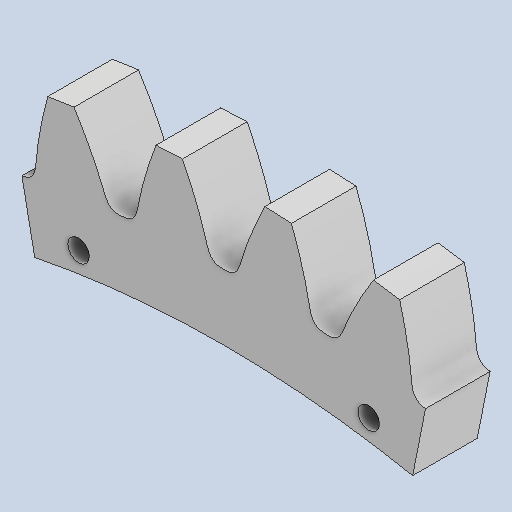
# Autodesk Inventor part: sector big gear
Saved by Autodesk Inventor 2025 (Build 290162010, 162A)
## iProperties
Created: 2025-08-27
Part Number: sector big gear
Material: Generic
Document SubType Name: Modeling
Designer: pokla
Density: 1 g/cm^3
Appearance: Default
Author: pokla
Autodesk Inventor part; units mm, degrees
(part 1 of 2)
ref_plane "YZ Plane" through (0, 0, 0) normal (1, 0, 0) x (0, 1, 0)
ref_plane "XZ Plane" through (0, 0, 0) normal (0, 1, 0) x (-1, 0, 0)
ref_plane "XY Plane" through (0, 0, 0) normal (0, 0, 1) x (1, 0, 0)
sketch "Sketch1" plane through (0, 0, 0) normal (0, 0, 1) x (1, 0, 0)
  spline S0 degree 3 poles (-15.3136, 412.2157) (-14.7005, 410.9627) (-13.4744, 408.4567) (-11.7613, 404.6382) (-10.1461, 400.7772) (-8.6557, 396.867) (-7.2691, 392.9165) (-6.406, 389.9001) (-5.7884, 387.899) (-5.3377, 386.951) (-4.8395, 386.2299) (-4.359, 385.7235) (-3.8332, 385.2647) (-3.236, 384.8928) (-2.5894, 384.6288) (-2.0848, 384.4891) (-1.5698, 384.3899) (-0.8714, 384.3654) (0, 384.3814) (0.8714, 384.3654) (1.5698, 384.3899) (2.0848, 384.4891) (2.5894, 384.6288) (3.236, 384.8928) (3.8332, 385.2647) (4.359, 385.7235) (4.8395, 386.2299) (5.3377, 386.951) (5.7884, 387.899) (6.406, 389.9001) (7.2691, 392.9165) (8.6557, 396.867) (10.1461, 400.7772) (11.7613, 404.6382) (13.4744, 408.4567) (14.7005, 410.9627) (15.3136, 412.2157) knots 0 0 0 0 0.418453 0.836906 1.255357 1.673806 2.09225 2.510695 2.615288 2.719831 2.824322 2.876636 2.92893 3.033403 3.085707 3.138007 3.190298 3.242598 3.347213 3.451829 3.504129 3.55642 3.60872 3.661023 3.765497 3.817791 3.870105 3.974596 4.079139 4.183732 4.602176 5.020621 5.43907 5.857521 6.275974 6.694427 6.694427 6.694427 6.694427
  circle A0 centre (0, 0) radius 384.375 construction
  circle A1 centre (0, 0) radius 375.877 construction
  circle A2 centre (0, 0) radius 400 construction
  circle A3 centre (0, 0) radius 412.5
  point P0 (-13.4954, 408.4468)
  point P1 (-11.7776, 404.6311)
  point P2 (-10.1669, 400.769)
  point P3 (-8.673, 396.8603)
  point P4 (-7.3084, 392.9046)
  point P5 (-6.0957, 388.8997)
  point P6 (-5.7647, 387.9075)
  point P7 (-5.3131, 386.9647)
  point P8 (-4.7127, 386.1094)
  point P9 (-4.3533, 385.7294)
  point P10 (-3.9585, 385.3864)
  point P11 (-3.0706, 384.8359)
  point P12 (-2.5862, 384.6385)
  point P13 (-2.083, 384.4958)
  point P14 (-1.5684, 384.4034)
  point P15 (-1.0462, 384.3746)
  point P16 (0, 384.375)
  point P17 (1.0462, 384.3746)
  point P18 (1.5684, 384.4034)
  point P19 (2.083, 384.4958)
  point P20 (2.5862, 384.6385)
  point P21 (3.0706, 384.8359)
  point P22 (3.9585, 385.3864)
  point P23 (4.3533, 385.7294)
  point P24 (4.7127, 386.1094)
  point P25 (5.3131, 386.9647)
  point P26 (5.7647, 387.9075)
  point P27 (6.0957, 388.8997)
  point P28 (7.3084, 392.9046)
  point P29 (8.673, 396.8603)
  point P30 (10.1669, 400.769)
  point P31 (11.7776, 404.6311)
  point P32 (13.4954, 408.4468)
  constraints: 4 centre point, 2 point on circle, 75 other
extrude "Extrusion1" add sketch "Sketch1" against normal blind 24
extrude "Extrusion2" cut sketch "Sketch1" against normal through all contours A3 S0 picked at (-1.5801, 403.5429)
pattern_circular "Circular Pattern1" count 64 over 360 about axis through (0, 0, -10) along (0, 0, 1) of "Extrusion2"
sketch "Sketch2" plane through (0, 0, 0) normal (0, 0, 1) x (1, 0, 0)
  arc A0 (25.1644, 411.7317) -> (15.3136, 412.2157) centre (0, 0) ccw projected
  arc A1 (-15.3136, 412.2157) -> (-25.1644, 411.7317) centre (0, 0) ccw projected
  arc A2 (-55.644, 408.7297) -> (-65.4, 407.2826) centre (0, 0) ccw projected
  spline S0 degree 3 poles (-65.4, 407.2826) (-65.7568, 405.9341) (-66.4705, 403.237) (-67.4057, 399.1577) (-68.2366, 395.0558) (-68.9355, 390.9299) (-69.5247, 386.7848) (-69.7828, 383.658) (-69.9982, 381.5749) (-70.2552, 380.5572) (-70.6032, 379.7528) (-70.9757, 379.1623) (-71.4018, 378.6098) (-71.915, 378.1285) (-72.4977, 377.7435) (-72.9654, 377.508) (-73.4511, 377.3102) (-74.1313, 377.1499) (-74.9891, 376.9957) (-75.8406, 376.8099) (-76.5304, 376.6977) (-77.0548, 376.6945) (-77.5771, 376.7331) (-78.2627, 376.8658) (-78.921, 377.1141) (-79.5261, 377.4615) (-80.0962, 377.8645) (-80.7256, 378.4745) (-81.3525, 379.3164) (-82.3487, 381.1585) (-83.7837, 383.9485) (-85.9143, 387.5526) (-88.1389, 391.097) (-90.4763, 394.5686) (-92.9014, 397.9796) (-94.5929, 400.1982) (-95.4386, 401.3075) knots 0 0 0 0 0.062508 0.125015 0.187523 0.25003 0.312536 0.375043 0.390666 0.406283 0.421892 0.429706 0.437518 0.453124 0.460937 0.468749 0.47656 0.484373 0.5 0.515627 0.52344 0.531251 0.539063 0.546876 0.562482 0.570294 0.578108 0.593717 0.609334 0.624957 0.687464 0.74997 0.812477 0.874985 0.937492 1 1 1 1 projected
  arc A3 (-95.4386, 401.3075) -> (-105.0057, 398.9111) centre (0, 0) ccw projected
  spline S1 degree 3 poles (-105.0057, 398.9111) (-105.2286, 397.5341) (-105.6745, 394.7801) (-106.2054, 390.6287) (-106.6303, 386.4651) (-106.9214, 382.2906) (-107.1015, 378.1077) (-107.0519, 374.9707) (-107.062, 372.8765) (-107.2181, 371.8385) (-107.4855, 371.0038) (-107.7983, 370.3797) (-108.1683, 369.7881) (-108.6318, 369.2588) (-109.1739, 368.8185) (-109.6163, 368.5383) (-110.0803, 368.2939) (-110.7415, 368.0677) (-111.58, 367.8301) (-112.4092, 367.5618) (-113.0847, 367.3825) (-113.6063, 367.3279) (-114.1298, 367.3152) (-114.8251, 367.38) (-115.5046, 367.5626) (-116.1409, 367.849) (-116.7477, 368.1942) (-117.4338, 368.7396) (-118.1403, 369.5159) (-119.3122, 371.2516) (-121.0137, 373.8875) (-123.4874, 377.2654) (-126.0487, 380.5746) (-128.7151, 383.8005) (-131.4629, 386.9573) (-133.3637, 388.9994) (-134.3141, 390.0205) knots 0 0 0 0 0.062508 0.125015 0.187523 0.25003 0.312536 0.375043 0.390666 0.406283 0.421892 0.429706 0.437518 0.453124 0.460937 0.468749 0.47656 0.484373 0.5 0.515627 0.52344 0.531251 0.539063 0.546876 0.562482 0.570294 0.578108 0.593717 0.609334 0.624957 0.687464 0.74997 0.812477 0.874985 0.937492 1 1 1 1 projected
  arc A4 (-134.3141, 390.0205) -> (-143.6002, 386.6979) centre (0, 0) ccw projected
  spline S2 degree 3 poles (-143.6002, 386.6979) (-143.6871, 385.3056) (-143.8609, 382.5212) (-143.9823, 378.3378) (-143.9971, 374.1526) (-143.8776, 369.9697) (-143.6468, 365.7892) (-143.2899, 362.6722) (-143.0948, 360.5871) (-143.1483, 359.5388) (-143.3327, 358.6819) (-143.5828, 358.0301) (-143.893, 357.4051) (-144.3024, 356.8329) (-144.7987, 356.3416) (-145.2115, 356.0194) (-145.6494, 355.7307) (-146.2852, 355.4408) (-147.0964, 355.1221) (-147.8953, 354.7738) (-148.55, 354.5292) (-149.0637, 354.4238) (-149.5834, 354.3598) (-150.2818, 354.3562) (-150.9759, 354.4713) (-151.6371, 354.6939) (-152.2749, 354.9779) (-153.0112, 355.4535) (-153.7903, 356.1568) (-155.1267, 357.7693) (-157.0784, 360.2257) (-159.8713, 363.3449) (-162.7446, 366.3871) (-165.7143, 369.3361) (-168.7583, 372.2083) (-170.8501, 374.0544) (-171.896, 374.9774) knots 0 0 0 0 0.062508 0.125015 0.187523 0.25003 0.312536 0.375043 0.390666 0.406283 0.421892 0.429706 0.437518 0.453124 0.460937 0.468749 0.47656 0.484373 0.5 0.515627 0.52344 0.531251 0.539063 0.546876 0.562482 0.570294 0.578108 0.593717 0.609334 0.624957 0.687464 0.74997 0.812477 0.874985 0.937492 1 1 1 1 projected
  arc A5 (-171.896, 374.9774) -> (-180.8117, 370.7605) centre (0, 0) ccw projected
  spline S3 degree 3 poles (-180.8117, 370.7605) (-180.7618, 369.3665) (-180.6618, 366.5784) (-180.3726, 362.4032) (-179.977, 358.2368) (-179.4481, 354.0857) (-178.8087, 349.948) (-178.1481, 346.881) (-177.7494, 344.825) (-177.7, 343.7765) (-177.7995, 342.9057) (-177.9845, 342.2325) (-178.2319, 341.5801) (-178.5833, 340.9705) (-179.0291, 340.433) (-179.4083, 340.0719) (-179.8157, 339.7416) (-180.4201, 339.3908) (-181.1962, 338.9942) (-181.9571, 338.5692) (-182.5846, 338.2616) (-183.0855, 338.1063) (-183.5965, 337.9917) (-184.2911, 337.9197) (-184.9931, 337.9662) (-185.673, 338.1229) (-186.3356, 338.3431) (-187.1149, 338.7442) (-187.9592, 339.3678) (-189.4472, 340.8414) (-191.6303, 343.0947) (-194.7155, 345.9252) (-197.8731, 348.6711) (-201.1176, 351.3148) (-204.4285, 353.8749) (-206.6912, 355.5069) (-207.8225, 356.323) knots 0 0 0 0 0.062508 0.125015 0.187523 0.25003 0.312536 0.375043 0.390666 0.406283 0.421892 0.429706 0.437518 0.453124 0.460937 0.468749 0.47656 0.484373 0.5 0.515627 0.52344 0.531251 0.539063 0.546876 0.562482 0.570294 0.578108 0.593717 0.609334 0.624957 0.687464 0.74997 0.812477 0.874985 0.937492 1 1 1 1 projected
  arc A6 (-207.8225, 356.323) -> (-216.282, 351.2526) centre (0, 0) ccw projected
  spline S4 degree 3 poles (-216.282, 351.2526) (-216.0956, 349.8701) (-215.7228, 347.1053) (-215.0258, 342.9785) (-214.2237, 338.8709) (-213.2905, 334.7917) (-212.2486, 330.7366) (-211.2905, 327.7491) (-210.6923, 325.7421) (-210.5403, 324.7035) (-210.554, 323.8271) (-210.6721, 323.139) (-210.8544, 322.4655) (-211.1443, 321.8245) (-211.5353, 321.2458) (-211.8773, 320.8492) (-212.2504, 320.4807) (-212.8174, 320.0722) (-213.5509, 319.6015) (-214.2665, 319.104) (-214.8608, 318.7364) (-215.3441, 318.5327) (-215.8414, 318.3686) (-216.5256, 318.2288) (-217.2288, 318.2063) (-217.9208, 318.2956) (-218.6017, 318.4498) (-219.4166, 318.7725) (-220.318, 319.3104) (-221.9433, 320.6311) (-224.3367, 322.6596) (-227.6844, 325.174) (-231.096, 327.5972) (-234.5841, 329.9101) (-238.1299, 332.1334) (-240.5417, 333.5358) (-241.7475, 334.237) knots 0 0 0 0 0.062508 0.125015 0.187523 0.25003 0.312536 0.375043 0.390666 0.406283 0.421892 0.429706 0.437518 0.453124 0.460937 0.468749 0.47656 0.484373 0.5 0.515627 0.52344 0.531251 0.539063 0.546876 0.562482 0.570294 0.578108 0.593717 0.609334 0.624957 0.687464 0.74997 0.812477 0.874985 0.937492 1 1 1 1 projected
  arc A7 (-241.7475, 334.237) -> (-249.6693, 328.3618) centre (0, 0) ccw projected
  spline S5 degree 3 poles (-249.6693, 328.3618) (-249.3483, 327.0043) (-248.7063, 324.2894) (-247.6081, 320.2508) (-246.4074, 316.2416) (-245.0788, 312.2735) (-243.6444, 308.34) (-242.3981, 305.4608) (-241.6061, 303.5221) (-241.353, 302.5034) (-241.2807, 301.6299) (-241.3308, 300.9336) (-241.4462, 300.2454) (-241.6719, 299.579) (-242.0043, 298.9648) (-242.3057, 298.5367) (-242.6409, 298.1333) (-243.1652, 297.6712) (-243.849, 297.1309) (-244.5124, 296.5656) (-245.0678, 296.1416) (-245.5289, 295.8915) (-246.0076, 295.6794) (-246.6748, 295.4732) (-247.3725, 295.3819) (-248.0699, 295.403) (-248.7627, 295.4896) (-249.6053, 295.731) (-250.555, 296.1779) (-252.3019, 297.3329) (-254.8827, 299.117) (-258.4607, 301.2912) (-262.0934, 303.3684) (-265.7913, 305.3283) (-269.538, 307.1932) (-272.0756, 308.3525) (-273.3444, 308.9322) knots 0 0 0 0 0.062508 0.125015 0.187523 0.25003 0.312536 0.375043 0.390666 0.406283 0.421892 0.429706 0.437518 0.453124 0.460937 0.468749 0.47656 0.484373 0.5 0.515627 0.52344 0.531251 0.539063 0.546876 0.562482 0.570294 0.578108 0.593717 0.609334 0.624957 0.687464 0.74997 0.812477 0.874985 0.937492 1 1 1 1 projected
  arc A8 (-273.3444, 308.9322) -> (-280.6521, 302.3088) centre (0, 0) ccw projected
  spline S6 degree 3 poles (-280.6521, 302.3088) (-280.1997, 300.9893) (-279.2947, 298.3503) (-277.8059, 294.4389) (-276.2179, 290.5667) (-274.5068, 286.7478) (-272.6938, 282.9739) (-271.1713, 280.2307) (-270.193, 278.379) (-269.8414, 277.39) (-269.6838, 276.5278) (-269.6654, 275.8299) (-269.7128, 275.1338) (-269.8721, 274.4485) (-270.1426, 273.8047) (-270.4007, 273.349) (-270.6947, 272.9147) (-271.1712, 272.4035) (-271.7987, 271.7987) (-272.4035, 271.1712) (-272.9147, 270.6947) (-273.349, 270.4007) (-273.8047, 270.1426) (-274.4485, 269.8721) (-275.1338, 269.7128) (-275.8299, 269.6654) (-276.5278, 269.6838) (-277.39, 269.8414) (-278.379, 270.193) (-280.2307, 271.1713) (-282.9739, 272.6938) (-286.7478, 274.5068) (-290.5667, 276.2179) (-294.4389, 277.8059) (-298.3503, 279.2947) (-300.9893, 280.1997) (-302.3088, 280.6521) knots 0 0 0 0 0.062508 0.125015 0.187523 0.25003 0.312536 0.375043 0.390666 0.406283 0.421892 0.429706 0.437518 0.453124 0.460937 0.468749 0.47656 0.484373 0.5 0.515627 0.52344 0.531251 0.539063 0.546876 0.562482 0.570294 0.578108 0.593717 0.609334 0.624957 0.687464 0.74997 0.812477 0.874985 0.937492 1 1 1 1 projected
  arc A9 (-302.3088, 280.6521) -> (-308.9322, 273.3444) centre (0, 0) ccw projected
  spline S7 degree 3 poles (-308.9322, 273.3444) (-308.3525, 272.0756) (-307.1932, 269.538) (-305.3283, 265.7913) (-303.3684, 262.0934) (-301.2912, 258.4607) (-299.117, 254.8827) (-297.3329, 252.3019) (-296.1779, 250.555) (-295.731, 249.6053) (-295.4896, 248.7627) (-295.403, 248.0699) (-295.3819, 247.3725) (-295.4732, 246.6748) (-295.6794, 246.0076) (-295.8915, 245.5289) (-296.1416, 245.0678) (-296.5656, 244.5124) (-297.1309, 243.849) (-297.6712, 243.1652) (-298.1333, 242.6409) (-298.5367, 242.3057) (-298.9648, 242.0043) (-299.579, 241.6719) (-300.2454, 241.4462) (-300.9336, 241.3308) (-301.6299, 241.2807) (-302.5034, 241.353) (-303.5221, 241.6061) (-305.4608, 242.3981) (-308.34, 243.6444) (-312.2735, 245.0788) (-316.2416, 246.4074) (-320.2508, 247.6081) (-324.2894, 248.7063) (-327.0043, 249.3483) (-328.3618, 249.6693) knots 0 0 0 0 0.062508 0.125015 0.187523 0.25003 0.312536 0.375043 0.390666 0.406283 0.421892 0.429706 0.437518 0.453124 0.460937 0.468749 0.47656 0.484373 0.5 0.515627 0.52344 0.531251 0.539063 0.546876 0.562482 0.570294 0.578108 0.593717 0.609334 0.624957 0.687464 0.74997 0.812477 0.874985 0.937492 1 1 1 1 projected
  arc A10 (-328.3618, 249.6693) -> (-334.237, 241.7475) centre (0, 0) ccw projected
  spline S8 degree 3 poles (-334.237, 241.7475) (-333.5358, 240.5417) (-332.1334, 238.1299) (-329.9101, 234.5841) (-327.5972, 231.096) (-325.174, 227.6844) (-322.6596, 224.3367) (-320.6311, 221.9433) (-319.3104, 220.318) (-318.7725, 219.4166) (-318.4498, 218.6017) (-318.2956, 217.9208) (-318.2063, 217.2288) (-318.2288, 216.5256) (-318.3686, 215.8414) (-318.5327, 215.3441) (-318.7364, 214.8608) (-319.104, 214.2665) (-319.6015, 213.5509) (-320.0722, 212.8174) (-320.4807, 212.2504) (-320.8492, 211.8773) (-321.2458, 211.5353) (-321.8245, 211.1443) (-322.4655, 210.8544) (-323.139, 210.6721) (-323.8271, 210.554) (-324.7035, 210.5403) (-325.7421, 210.6923) (-327.7491, 211.2905) (-330.7366, 212.2486) (-334.7917, 213.2905) (-338.8709, 214.2237) (-342.9785, 215.0258) (-347.1053, 215.7228) (-349.8701, 216.0956) (-351.2526, 216.282) knots 0 0 0 0 0.062508 0.125015 0.187523 0.25003 0.312536 0.375043 0.390666 0.406283 0.421892 0.429706 0.437518 0.453124 0.460937 0.468749 0.47656 0.484373 0.5 0.515627 0.52344 0.531251 0.539063 0.546876 0.562482 0.570294 0.578108 0.593717 0.609334 0.624957 0.687464 0.74997 0.812477 0.874985 0.937492 1 1 1 1 projected
  arc A11 (-351.2526, 216.282) -> (-356.323, 207.8225) centre (0, 0) ccw projected
  spline S9 degree 3 poles (-356.323, 207.8225) (-355.5069, 206.6912) (-353.8749, 204.4285) (-351.3148, 201.1176) (-348.6711, 197.8731) (-345.9252, 194.7155) (-343.0947, 191.6303) (-340.8414, 189.4472) (-339.3678, 187.9592) (-338.7442, 187.1149) (-338.3431, 186.3356) (-338.1229, 185.673) (-337.9662, 184.9931) (-337.9197, 184.2911) (-337.9917, 183.5965) (-338.1063, 183.0855) (-338.2616, 182.5846) (-338.5692, 181.9571) (-338.9942, 181.1962) (-339.3908, 180.4201) (-339.7416, 179.8157) (-340.0719, 179.4083) (-340.433, 179.0291) (-340.9705, 178.5833) (-341.5801, 178.2319) (-342.2325, 177.9845) (-342.9057, 177.7995) (-343.7765, 177.7) (-344.825, 177.7494) (-346.881, 178.1481) (-349.948, 178.8087) (-354.0857, 179.4481) (-358.2368, 179.977) (-362.4032, 180.3726) (-366.5784, 180.6618) (-369.3665, 180.7618) (-370.7605, 180.8117) knots 0 0 0 0 0.062508 0.125015 0.187523 0.25003 0.312536 0.375043 0.390666 0.406283 0.421892 0.429706 0.437518 0.453124 0.460937 0.468749 0.47656 0.484373 0.5 0.515627 0.52344 0.531251 0.539063 0.546876 0.562482 0.570294 0.578108 0.593717 0.609334 0.624957 0.687464 0.74997 0.812477 0.874985 0.937492 1 1 1 1 projected
  arc A12 (-370.7605, 180.8117) -> (-374.9774, 171.896) centre (0, 0) ccw projected
  spline S10 degree 3 poles (-374.9774, 171.896) (-374.0544, 170.8501) (-372.2083, 168.7583) (-369.3361, 165.7143) (-366.3871, 162.7446) (-363.3449, 159.8713) (-360.2257, 157.0784) (-357.7693, 155.1267) (-356.1568, 153.7903) (-355.4535, 153.0112) (-354.9779, 152.2749) (-354.6939, 151.6371) (-354.4713, 150.9759) (-354.3562, 150.2818) (-354.3598, 149.5834) (-354.4238, 149.0637) (-354.5292, 148.55) (-354.7738, 147.8953) (-355.1221, 147.0964) (-355.4408, 146.2852) (-355.7307, 145.6494) (-356.0194, 145.2115) (-356.3416, 144.7987) (-356.8329, 144.3024) (-357.4051, 143.893) (-358.0301, 143.5828) (-358.6819, 143.3327) (-359.5388, 143.1483) (-360.5871, 143.0948) (-362.6722, 143.2899) (-365.7892, 143.6468) (-369.9697, 143.8776) (-374.1526, 143.9971) (-378.3378, 143.9823) (-382.5212, 143.8609) (-385.3056, 143.6871) (-386.6979, 143.6002) knots 0 0 0 0 0.062508 0.125015 0.187523 0.25003 0.312536 0.375043 0.390666 0.406283 0.421892 0.429706 0.437518 0.453124 0.460937 0.468749 0.47656 0.484373 0.5 0.515627 0.52344 0.531251 0.539063 0.546876 0.562482 0.570294 0.578108 0.593717 0.609334 0.624957 0.687464 0.74997 0.812477 0.874985 0.937492 1 1 1 1 projected
  arc A13 (-386.6979, 143.6002) -> (-390.0205, 134.3141) centre (0, 0) ccw projected
  spline S11 degree 3 poles (-390.0205, 134.3141) (-388.9994, 133.3637) (-386.9573, 131.4629) (-383.8005, 128.7151) (-380.5746, 126.0487) (-377.2654, 123.4874) (-373.8875, 121.0137) (-371.2516, 119.3122) (-369.5159, 118.1403) (-368.7396, 117.4338) (-368.1942, 116.7477) (-367.849, 116.1409) (-367.5626, 115.5046) (-367.38, 114.8251) (-367.3152, 114.1298) (-367.3279, 113.6063) (-367.3825, 113.0847) (-367.5618, 112.4092) (-367.8301, 111.58) (-368.0677, 110.7415) (-368.2939, 110.0803) (-368.5383, 109.6163) (-368.8185, 109.1739) (-369.2588, 108.6318) (-369.7881, 108.1683) (-370.3797, 107.7983) (-371.0038, 107.4855) (-371.8385, 107.2181) (-372.8765, 107.062) (-374.9707, 107.0519) (-378.1077, 107.1015) (-382.2906, 106.9214) (-386.4651, 106.6303) (-390.6287, 106.2054) (-394.7801, 105.6745) (-397.5341, 105.2286) (-398.9111, 105.0057) knots 0 0 0 0 0.062508 0.125015 0.187523 0.25003 0.312536 0.375043 0.390666 0.406283 0.421892 0.429706 0.437518 0.453124 0.460937 0.468749 0.47656 0.484373 0.5 0.515627 0.52344 0.531251 0.539063 0.546876 0.562482 0.570294 0.578108 0.593717 0.609334 0.624957 0.687464 0.74997 0.812477 0.874985 0.937492 1 1 1 1 projected
  arc A14 (-398.9111, 105.0057) -> (-401.3075, 95.4386) centre (0, 0) ccw projected
  spline S12 degree 3 poles (-401.3075, 95.4386) (-400.1982, 94.5929) (-397.9796, 92.9014) (-394.5686, 90.4763) (-391.097, 88.1389) (-387.5526, 85.9143) (-383.9485, 83.7837) (-381.1585, 82.3487) (-379.3164, 81.3525) (-378.4745, 80.7256) (-377.8645, 80.0962) (-377.4615, 79.5261) (-377.1141, 78.921) (-376.8658, 78.2627) (-376.7331, 77.5771) (-376.6945, 77.0548) (-376.6977, 76.5304) (-376.8099, 75.8406) (-376.9957, 74.9891) (-377.1499, 74.1313) (-377.3102, 73.4511) (-377.508, 72.9654) (-377.7435, 72.4977) (-378.1285, 71.915) (-378.6098, 71.4018) (-379.1623, 70.9757) (-379.7528, 70.6032) (-380.5572, 70.2552) (-381.5749, 69.9982) (-383.658, 69.7828) (-386.7848, 69.5247) (-390.9299, 68.9355) (-395.0558, 68.2366) (-399.1577, 67.4057) (-403.237, 66.4705) (-405.9341, 65.7568) (-407.2826, 65.4) knots 0 0 0 0 0.062508 0.125015 0.187523 0.25003 0.312536 0.375043 0.390666 0.406283 0.421892 0.429706 0.437518 0.453124 0.460937 0.468749 0.47656 0.484373 0.5 0.515627 0.52344 0.531251 0.539063 0.546876 0.562482 0.570294 0.578108 0.593717 0.609334 0.624957 0.687464 0.74997 0.812477 0.874985 0.937492 1 1 1 1 projected
  arc A15 (-407.2826, 65.4) -> (-408.7297, 55.644) centre (0, 0) ccw projected
  spline S13 degree 3 poles (-408.7297, 55.644) (-407.5429, 54.9111) (-405.1691, 53.4453) (-401.5369, 51.3661) (-397.8529, 49.3803) (-394.1076, 47.5138) (-390.312, 45.7467) (-387.3947, 44.5921) (-385.4638, 43.7813) (-384.5646, 43.2399) (-383.8958, 42.6733) (-383.4388, 42.1455) (-383.0338, 41.5773) (-382.7222, 40.9465) (-382.5229, 40.2772) (-382.4333, 39.7613) (-382.3851, 39.239) (-382.4291, 38.5416) (-382.5305, 37.676) (-382.5999, 36.8072) (-382.6928, 36.1146) (-382.842, 35.6118) (-383.0305, 35.1232) (-383.3566, 34.5057) (-383.7853, 33.9478) (-384.2933, 33.4695) (-384.8445, 33.041) (-385.611, 32.6158) (-386.5985, 32.2602) (-388.6505, 31.8417) (-391.7369, 31.2784) (-395.8044, 30.2857) (-399.8419, 29.1858) (-403.8425, 27.9568) (-407.8106, 26.6262) (-410.4247, 25.6517) (-411.7317, 25.1644) knots 0 0 0 0 0.062508 0.125015 0.187523 0.25003 0.312536 0.375043 0.390666 0.406283 0.421892 0.429706 0.437518 0.453124 0.460937 0.468749 0.47656 0.484373 0.5 0.515627 0.52344 0.531251 0.539063 0.546876 0.562482 0.570294 0.578108 0.593717 0.609334 0.624957 0.687464 0.74997 0.812477 0.874985 0.937492 1 1 1 1 projected
  arc A16 (-411.7317, 25.1644) -> (-412.2157, 15.3136) centre (0, 0) ccw projected
  spline S14 degree 3 poles (-412.2157, 15.3136) (-410.9627, 14.7005) (-408.4567, 13.4744) (-404.6382, 11.7613) (-400.7772, 10.1461) (-396.867, 8.6557) (-392.9165, 7.2691) (-389.9001, 6.406) (-387.899, 5.7884) (-386.951, 5.3377) (-386.2299, 4.8395) (-385.7235, 4.359) (-385.2647, 3.8332) (-384.8928, 3.236) (-384.6288, 2.5894) (-384.4891, 2.0848) (-384.3899, 1.5698) (-384.3654, 0.8714) (-384.3814, 0) (-384.3654, -0.8714) (-384.3899, -1.5698) (-384.4891, -2.0848) (-384.6288, -2.5894) (-384.8928, -3.236) (-385.2647, -3.8332) (-385.7235, -4.359) (-386.2299, -4.8395) (-386.951, -5.3377) (-387.899, -5.7884) (-389.9001, -6.406) (-392.9165, -7.2691) (-396.867, -8.6557) (-400.7772, -10.1461) (-404.6382, -11.7613) (-408.4567, -13.4744) (-410.9627, -14.7005) (-412.2157, -15.3136) knots 0 0 0 0 0.062508 0.125015 0.187523 0.25003 0.312536 0.375043 0.390666 0.406283 0.421892 0.429706 0.437518 0.453124 0.460937 0.468749 0.47656 0.484373 0.5 0.515627 0.52344 0.531251 0.539063 0.546876 0.562482 0.570294 0.578108 0.593717 0.609334 0.624957 0.687464 0.74997 0.812477 0.874985 0.937492 1 1 1 1 projected
  arc A17 (-412.2157, -15.3136) -> (-411.7317, -25.1644) centre (0, 0) ccw projected
  spline S15 degree 3 poles (-411.7317, -25.1644) (-410.4247, -25.6517) (-407.8106, -26.6262) (-403.8425, -27.9568) (-399.8419, -29.1858) (-395.8044, -30.2857) (-391.7369, -31.2784) (-388.6505, -31.8417) (-386.5985, -32.2602) (-385.611, -32.6158) (-384.8445, -33.041) (-384.2933, -33.4695) (-383.7853, -33.9478) (-383.3566, -34.5057) (-383.0305, -35.1232) (-382.842, -35.6118) (-382.6928, -36.1146) (-382.5999, -36.8072) (-382.5305, -37.676) (-382.4291, -38.5416) (-382.3851, -39.239) (-382.4333, -39.7613) (-382.5229, -40.2772) (-382.7222, -40.9465) (-383.0338, -41.5773) (-383.4388, -42.1455) (-383.8958, -42.6733) (-384.5646, -43.2399) (-385.4638, -43.7813) (-387.3947, -44.5921) (-390.312, -45.7467) (-394.1076, -47.5138) (-397.8529, -49.3803) (-401.5369, -51.3661) (-405.1691, -53.4453) (-407.5429, -54.9111) (-408.7297, -55.644) knots 0 0 0 0 0.062508 0.125015 0.187523 0.25003 0.312536 0.375043 0.390666 0.406283 0.421892 0.429706 0.437518 0.453124 0.460937 0.468749 0.47656 0.484373 0.5 0.515627 0.52344 0.531251 0.539063 0.546876 0.562482 0.570294 0.578108 0.593717 0.609334 0.624957 0.687464 0.74997 0.812477 0.874985 0.937492 1 1 1 1 projected
  arc A18 (-408.7297, -55.644) -> (-407.2826, -65.4) centre (0, 0) ccw projected
  spline S16 degree 3 poles (-407.2826, -65.4) (-405.9341, -65.7568) (-403.237, -66.4705) (-399.1577, -67.4057) (-395.0558, -68.2366) (-390.9299, -68.9355) (-386.7848, -69.5247) (-383.658, -69.7828) (-381.5749, -69.9982) (-380.5572, -70.2552) (-379.7528, -70.6032) (-379.1623, -70.9757) (-378.6098, -71.4018) (-378.1285, -71.915) (-377.7435, -72.4977) (-377.508, -72.9654) (-377.3102, -73.4511) (-377.1499, -74.1313) (-376.9957, -74.9891) (-376.8099, -75.8406) (-376.6977, -76.5304) (-376.6945, -77.0548) (-376.7331, -77.5771) (-376.8658, -78.2627) (-377.1141, -78.921) (-377.4615, -79.5261) (-377.8645, -80.0962) (-378.4745, -80.7256) (-379.3164, -81.3525) (-381.1585, -82.3487) (-383.9485, -83.7837) (-387.5526, -85.9143) (-391.097, -88.1389) (-394.5686, -90.4763) (-397.9796, -92.9014) (-400.1982, -94.5929) (-401.3075, -95.4386) knots 0 0 0 0 0.062508 0.125015 0.187523 0.25003 0.312536 0.375043 0.390666 0.406283 0.421892 0.429706 0.437518 0.453124 0.460937 0.468749 0.47656 0.484373 0.5 0.515627 0.52344 0.531251 0.539063 0.546876 0.562482 0.570294 0.578108 0.593717 0.609334 0.624957 0.687464 0.74997 0.812477 0.874985 0.937492 1 1 1 1 projected
  arc A19 (-401.3075, -95.4386) -> (-398.9111, -105.0057) centre (0, 0) ccw projected
  spline S17 degree 3 poles (-398.9111, -105.0057) (-397.5341, -105.2286) (-394.7801, -105.6745) (-390.6287, -106.2054) (-386.4651, -106.6303) (-382.2906, -106.9214) (-378.1077, -107.1015) (-374.9707, -107.0519) (-372.8765, -107.062) (-371.8385, -107.2181) (-371.0038, -107.4855) (-370.3797, -107.7983) (-369.7881, -108.1683) (-369.2588, -108.6318) (-368.8185, -109.1739) (-368.5383, -109.6163) (-368.2939, -110.0803) (-368.0677, -110.7415) (-367.8301, -111.58) (-367.5618, -112.4092) (-367.3825, -113.0847) (-367.3279, -113.6063) (-367.3152, -114.1298) (-367.38, -114.8251) (-367.5626, -115.5046) (-367.849, -116.1409) (-368.1942, -116.7477) (-368.7396, -117.4338) (-369.5159, -118.1403) (-371.2516, -119.3122) (-373.8875, -121.0137) (-377.2654, -123.4874) (-380.5746, -126.0487) (-383.8005, -128.7151) (-386.9573, -131.4629) (-388.9994, -133.3637) (-390.0205, -134.3141) knots 0 0 0 0 0.062508 0.125015 0.187523 0.25003 0.312536 0.375043 0.390666 0.406283 0.421892 0.429706 0.437518 0.453124 0.460937 0.468749 0.47656 0.484373 0.5 0.515627 0.52344 0.531251 0.539063 0.546876 0.562482 0.570294 0.578108 0.593717 0.609334 0.624957 0.687464 0.74997 0.812477 0.874985 0.937492 1 1 1 1 projected
  arc A20 (-390.0205, -134.3141) -> (-386.6979, -143.6002) centre (0, 0) ccw projected
  spline S18 degree 3 poles (-386.6979, -143.6002) (-385.3056, -143.6871) (-382.5212, -143.8609) (-378.3378, -143.9823) (-374.1526, -143.9971) (-369.9697, -143.8776) (-365.7892, -143.6468) (-362.6722, -143.2899) (-360.5871, -143.0948) (-359.5388, -143.1483) (-358.6819, -143.3327) (-358.0301, -143.5828) (-357.4051, -143.893) (-356.8329, -144.3024) (-356.3416, -144.7987) (-356.0194, -145.2115) (-355.7307, -145.6494) (-355.4408, -146.2852) (-355.1221, -147.0964) (-354.7738, -147.8953) (-354.5292, -148.55) (-354.4238, -149.0637) (-354.3598, -149.5834) (-354.3562, -150.2818) (-354.4713, -150.9759) (-354.6939, -151.6371) (-354.9779, -152.2749) (-355.4535, -153.0112) (-356.1568, -153.7903) (-357.7693, -155.1267) (-360.2257, -157.0784) (-363.3449, -159.8713) (-366.3871, -162.7446) (-369.3361, -165.7143) (-372.2083, -168.7583) (-374.0544, -170.8501) (-374.9774, -171.896) knots 0 0 0 0 0.062508 0.125015 0.187523 0.25003 0.312536 0.375043 0.390666 0.406283 0.421892 0.429706 0.437518 0.453124 0.460937 0.468749 0.47656 0.484373 0.5 0.515627 0.52344 0.531251 0.539063 0.546876 0.562482 0.570294 0.578108 0.593717 0.609334 0.624957 0.687464 0.74997 0.812477 0.874985 0.937492 1 1 1 1 projected
  arc A21 (-374.9774, -171.896) -> (-370.7605, -180.8117) centre (0, 0) ccw projected
  spline S19 degree 3 poles (-370.7605, -180.8117) (-369.3665, -180.7618) (-366.5784, -180.6618) (-362.4032, -180.3726) (-358.2368, -179.977) (-354.0857, -179.4481) (-349.948, -178.8087) (-346.881, -178.1481) (-344.825, -177.7494) (-343.7765, -177.7) (-342.9057, -177.7995) (-342.2325, -177.9845) (-341.5801, -178.2319) (-340.9705, -178.5833) (-340.433, -179.0291) (-340.0719, -179.4083) (-339.7416, -179.8157) (-339.3908, -180.4201) (-338.9942, -181.1962) (-338.5692, -181.9571) (-338.2616, -182.5846) (-338.1063, -183.0855) (-337.9917, -183.5965) (-337.9197, -184.2911) (-337.9662, -184.9931) (-338.1229, -185.673) (-338.3431, -186.3356) (-338.7442, -187.1149) (-339.3678, -187.9592) (-340.8414, -189.4472) (-343.0947, -191.6303) (-345.9252, -194.7155) (-348.6711, -197.8731) (-351.3148, -201.1176) (-353.8749, -204.4285) (-355.5069, -206.6912) (-356.323, -207.8225) knots 0 0 0 0 0.062508 0.125015 0.187523 0.25003 0.312536 0.375043 0.390666 0.406283 0.421892 0.429706 0.437518 0.453124 0.460937 0.468749 0.47656 0.484373 0.5 0.515627 0.52344 0.531251 0.539063 0.546876 0.562482 0.570294 0.578108 0.593717 0.609334 0.624957 0.687464 0.74997 0.812477 0.874985 0.937492 1 1 1 1 projected
  arc A22 (-356.323, -207.8225) -> (-351.2526, -216.282) centre (0, 0) ccw projected
  spline S20 degree 3 poles (-351.2526, -216.282) (-349.8701, -216.0956) (-347.1053, -215.7228) (-342.9785, -215.0258) (-338.8709, -214.2237) (-334.7917, -213.2905) (-330.7366, -212.2486) (-327.7491, -211.2905) (-325.7421, -210.6923) (-324.7035, -210.5403) (-323.8271, -210.554) (-323.139, -210.6721) (-322.4655, -210.8544) (-321.8245, -211.1443) (-321.2458, -211.5353) (-320.8492, -211.8773) (-320.4807, -212.2504) (-320.0722, -212.8174) (-319.6015, -213.5509) (-319.104, -214.2665) (-318.7364, -214.8608) (-318.5327, -215.3441) (-318.3686, -215.8414) (-318.2288, -216.5256) (-318.2063, -217.2288) (-318.2956, -217.9208) (-318.4498, -218.6017) (-318.7725, -219.4166) (-319.3104, -220.318) (-320.6311, -221.9433) (-322.6596, -224.3367) (-325.174, -227.6844) (-327.5972, -231.096) (-329.9101, -234.5841) (-332.1334, -238.1299) (-333.5358, -240.5417) (-334.237, -241.7475) knots 0 0 0 0 0.062508 0.125015 0.187523 0.25003 0.312536 0.375043 0.390666 0.406283 0.421892 0.429706 0.437518 0.453124 0.460937 0.468749 0.47656 0.484373 0.5 0.515627 0.52344 0.531251 0.539063 0.546876 0.562482 0.570294 0.578108 0.593717 0.609334 0.624957 0.687464 0.74997 0.812477 0.874985 0.937492 1 1 1 1 projected
  arc A23 (-334.237, -241.7475) -> (-328.3618, -249.6693) centre (0, 0) ccw projected
  spline S21 degree 3 poles (-328.3618, -249.6693) (-327.0043, -249.3483) (-324.2894, -248.7063) (-320.2508, -247.6081) (-316.2416, -246.4074) (-312.2735, -245.0788) (-308.34, -243.6444) (-305.4608, -242.3981) (-303.5221, -241.6061) (-302.5034, -241.353) (-301.6299, -241.2807) (-300.9336, -241.3308) (-300.2454, -241.4462) (-299.579, -241.6719) (-298.9648, -242.0043) (-298.5367, -242.3057) (-298.1333, -242.6409) (-297.6712, -243.1652) (-297.1309, -243.849) (-296.5656, -244.5124) (-296.1416, -245.0678) (-295.8915, -245.5289) (-295.6794, -246.0076) (-295.4732, -246.6748) (-295.3819, -247.3725) (-295.403, -248.0699) (-295.4896, -248.7627) (-295.731, -249.6053) (-296.1779, -250.555) (-297.3329, -252.3019) (-299.117, -254.8827) (-301.2912, -258.4607) (-303.3684, -262.0934) (-305.3283, -265.7913) (-307.1932, -269.538) (-308.3525, -272.0756) (-308.9322, -273.3444) knots 0 0 0 0 0.062508 0.125015 0.187523 0.25003 0.312536 0.375043 0.390666 0.406283 0.421892 0.429706 0.437518 0.453124 0.460937 0.468749 0.47656 0.484373 0.5 0.515627 0.52344 0.531251 0.539063 0.546876 0.562482 0.570294 0.578108 0.593717 0.609334 0.624957 0.687464 0.74997 0.812477 0.874985 0.937492 1 1 1 1 projected
  arc A24 (-308.9322, -273.3444) -> (-302.3088, -280.6521) centre (0, 0) ccw projected
  spline S22 degree 3 poles (-302.3088, -280.6521) (-300.9893, -280.1997) (-298.3503, -279.2947) (-294.4389, -277.8059) (-290.5667, -276.2179) (-286.7478, -274.5068) (-282.9739, -272.6938) (-280.2307, -271.1713) (-278.379, -270.193) (-277.39, -269.8414) (-276.5278, -269.6838) (-275.8299, -269.6654) (-275.1338, -269.7128) (-274.4485, -269.8721) (-273.8047, -270.1426) (-273.349, -270.4007) (-272.9147, -270.6947) (-272.4035, -271.1712) (-271.7987, -271.7987) (-271.1712, -272.4035) (-270.6947, -272.9147) (-270.4007, -273.349) (-270.1426, -273.8047) (-269.8721, -274.4485) (-269.7128, -275.1338) (-269.6654, -275.8299) (-269.6838, -276.5278) (-269.8414, -277.39) (-270.193, -278.379) (-271.1713, -280.2307) (-272.6938, -282.9739) (-274.5068, -286.7478) (-276.2179, -290.5667) (-277.8059, -294.4389) (-279.2947, -298.3503) (-280.1997, -300.9893) (-280.6521, -302.3088) knots 0 0 0 0 0.062508 0.125015 0.187523 0.25003 0.312536 0.375043 0.390666 0.406283 0.421892 0.429706 0.437518 0.453124 0.460937 0.468749 0.47656 0.484373 0.5 0.515627 0.52344 0.531251 0.539063 0.546876 0.562482 0.570294 0.578108 0.593717 0.609334 0.624957 0.687464 0.74997 0.812477 0.874985 0.937492 1 1 1 1 projected
  arc A25 (-280.6521, -302.3088) -> (-273.3444, -308.9322) centre (0, 0) ccw projected
  spline S23 degree 3 poles (-273.3444, -308.9322) (-272.0756, -308.3525) (-269.538, -307.1932) (-265.7913, -305.3283) (-262.0934, -303.3684) (-258.4607, -301.2912) (-254.8827, -299.117) (-252.3019, -297.3329) (-250.555, -296.1779) (-249.6053, -295.731) (-248.7627, -295.4896) (-248.0699, -295.403) (-247.3725, -295.3819) (-246.6748, -295.4732) (-246.0076, -295.6794) (-245.5289, -295.8915) (-245.0678, -296.1416) (-244.5124, -296.5656) (-243.849, -297.1309) (-243.1652, -297.6712) (-242.6409, -298.1333) (-242.3057, -298.5367) (-242.0043, -298.9648) (-241.6719, -299.579) (-241.4462, -300.2454) (-241.3308, -300.9336) (-241.2807, -301.6299) (-241.353, -302.5034) (-241.6061, -303.5221) (-242.3981, -305.4608) (-243.6444, -308.34) (-245.0788, -312.2735) (-246.4074, -316.2416) (-247.6081, -320.2508) (-248.7063, -324.2894) (-249.3483, -327.0043) (-249.6693, -328.3618) knots 0 0 0 0 0.062508 0.125015 0.187523 0.25003 0.312536 0.375043 0.390666 0.406283 0.421892 0.429706 0.437518 0.453124 0.460937 0.468749 0.47656 0.484373 0.5 0.515627 0.52344 0.531251 0.539063 0.546876 0.562482 0.570294 0.578108 0.593717 0.609334 0.624957 0.687464 0.74997 0.812477 0.874985 0.937492 1 1 1 1 projected
  arc A26 (-249.6693, -328.3618) -> (-241.7475, -334.237) centre (0, 0) ccw projected
  spline S24 degree 3 poles (-241.7475, -334.237) (-240.5417, -333.5358) (-238.1299, -332.1334) (-234.5841, -329.9101) (-231.096, -327.5972) (-227.6844, -325.174) (-224.3367, -322.6596) (-221.9433, -320.6311) (-220.318, -319.3104) (-219.4166, -318.7725) (-218.6017, -318.4498) (-217.9208, -318.2956) (-217.2288, -318.2063) (-216.5256, -318.2288) (-215.8414, -318.3686) (-215.3441, -318.5327) (-214.8608, -318.7364) (-214.2665, -319.104) (-213.5509, -319.6015) (-212.8174, -320.0722) (-212.2504, -320.4807) (-211.8773, -320.8492) (-211.5353, -321.2458) (-211.1443, -321.8245) (-210.8544, -322.4655) (-210.6721, -323.139) (-210.554, -323.8271) (-210.5403, -324.7035) (-210.6923, -325.7421) (-211.2905, -327.7491) (-212.2486, -330.7366) (-213.2905, -334.7917) (-214.2237, -338.8709) (-215.0258, -342.9785) (-215.7228, -347.1053) (-216.0956, -349.8701) (-216.282, -351.2526) knots 0 0 0 0 0.062508 0.125015 0.187523 0.25003 0.312536 0.375043 0.390666 0.406283 0.421892 0.429706 0.437518 0.453124 0.460937 0.468749 0.47656 0.484373 0.5 0.515627 0.52344 0.531251 0.539063 0.546876 0.562482 0.570294 0.578108 0.593717 0.609334 0.624957 0.687464 0.74997 0.812477 0.874985 0.937492 1 1 1 1 projected
  arc A27 (-216.282, -351.2526) -> (-207.8225, -356.323) centre (0, 0) ccw projected
  spline S25 degree 3 poles (-207.8225, -356.323) (-206.6912, -355.5069) (-204.4285, -353.8749) (-201.1176, -351.3148) (-197.8731, -348.6711) (-194.7155, -345.9252) (-191.6303, -343.0947) (-189.4472, -340.8414) (-187.9592, -339.3678) (-187.1149, -338.7442) (-186.3356, -338.3431) (-185.673, -338.1229) (-184.9931, -337.9662) (-184.2911, -337.9197) (-183.5965, -337.9917) (-183.0855, -338.1063) (-182.5846, -338.2616) (-181.9571, -338.5692) (-181.1962, -338.9942) (-180.4201, -339.3908) (-179.8157, -339.7416) (-179.4083, -340.0719) (-179.0291, -340.433) (-178.5833, -340.9705) (-178.2319, -341.5801) (-177.9845, -342.2325) (-177.7995, -342.9057) (-177.7, -343.7765) (-177.7494, -344.825) (-178.1481, -346.881) (-178.8087, -349.948) (-179.4481, -354.0857) (-179.977, -358.2368) (-180.3726, -362.4032) (-180.6618, -366.5784) (-180.7618, -369.3665) (-180.8117, -370.7605) knots 0 0 0 0 0.062508 0.125015 0.187523 0.25003 0.312536 0.375043 0.390666 0.406283 0.421892 0.429706 0.437518 0.453124 0.460937 0.468749 0.47656 0.484373 0.5 0.515627 0.52344 0.531251 0.539063 0.546876 0.562482 0.570294 0.578108 0.593717 0.609334 0.624957 0.687464 0.74997 0.812477 0.874985 0.937492 1 1 1 1 projected
  arc A28 (-180.8117, -370.7605) -> (-171.896, -374.9774) centre (0, 0) ccw projected
  spline S26 degree 3 poles (-171.896, -374.9774) (-170.8501, -374.0544) (-168.7583, -372.2083) (-165.7143, -369.3361) (-162.7446, -366.3871) (-159.8713, -363.3449) (-157.0784, -360.2257) (-155.1267, -357.7693) (-153.7903, -356.1568) (-153.0112, -355.4535) (-152.2749, -354.9779) (-151.6371, -354.6939) (-150.9759, -354.4713) (-150.2818, -354.3562) (-149.5834, -354.3598) (-149.0637, -354.4238) (-148.55, -354.5292) (-147.8953, -354.7738) (-147.0964, -355.1221) (-146.2852, -355.4408) (-145.6494, -355.7307) (-145.2115, -356.0194) (-144.7987, -356.3416) (-144.3024, -356.8329) (-143.893, -357.4051) (-143.5828, -358.0301) (-143.3327, -358.6819) (-143.1483, -359.5388) (-143.0948, -360.5871) (-143.2899, -362.6722) (-143.6468, -365.7892) (-143.8776, -369.9697) (-143.9971, -374.1526) (-143.9823, -378.3378) (-143.8609, -382.5212) (-143.6871, -385.3056) (-143.6002, -386.6979) knots 0 0 0 0 0.062508 0.125015 0.187523 0.25003 0.312536 0.375043 0.390666 0.406283 0.421892 0.429706 0.437518 0.453124 0.460937 0.468749 0.47656 0.484373 0.5 0.515627 0.52344 0.531251 0.539063 0.546876 0.562482 0.570294 0.578108 0.593717 0.609334 0.624957 0.687464 0.74997 0.812477 0.874985 0.937492 1 1 1 1 projected
  arc A29 (-143.6002, -386.6979) -> (-134.3141, -390.0205) centre (0, 0) ccw projected
  spline S27 degree 3 poles (-134.3141, -390.0205) (-133.3637, -388.9994) (-131.4629, -386.9573) (-128.7151, -383.8005) (-126.0487, -380.5746) (-123.4874, -377.2654) (-121.0137, -373.8875) (-119.3122, -371.2516) (-118.1403, -369.5159) (-117.4338, -368.7396) (-116.7477, -368.1942) (-116.1409, -367.849) (-115.5046, -367.5626) (-114.8251, -367.38) (-114.1298, -367.3152) (-113.6063, -367.3279) (-113.0847, -367.3825) (-112.4092, -367.5618) (-111.58, -367.8301) (-110.7415, -368.0677) (-110.0803, -368.2939) (-109.6163, -368.5383) (-109.1739, -368.8185) (-108.6318, -369.2588) (-108.1683, -369.7881) (-107.7983, -370.3797) (-107.4855, -371.0038) (-107.2181, -371.8385) (-107.062, -372.8765) (-107.0519, -374.9707) (-107.1015, -378.1077) (-106.9214, -382.2906) (-106.6303, -386.4651) (-106.2054, -390.6287) (-105.6745, -394.7801) (-105.2286, -397.5341) (-105.0057, -398.9111) knots 0 0 0 0 0.062508 0.125015 0.187523 0.25003 0.312536 0.375043 0.390666 0.406283 0.421892 0.429706 0.437518 0.453124 0.460937 0.468749 0.47656 0.484373 0.5 0.515627 0.52344 0.531251 0.539063 0.546876 0.562482 0.570294 0.578108 0.593717 0.609334 0.624957 0.687464 0.74997 0.812477 0.874985 0.937492 1 1 1 1 projected
  arc A30 (-105.0057, -398.9111) -> (-95.4386, -401.3075) centre (0, 0) ccw projected
  spline S28 degree 3 poles (-95.4386, -401.3075) (-94.5929, -400.1982) (-92.9014, -397.9796) (-90.4763, -394.5686) (-88.1389, -391.097) (-85.9143, -387.5526) (-83.7837, -383.9485) (-82.3487, -381.1585) (-81.3525, -379.3164) (-80.7256, -378.4745) (-80.0962, -377.8645) (-79.5261, -377.4615) (-78.921, -377.1141) (-78.2627, -376.8658) (-77.5771, -376.7331) (-77.0548, -376.6945) (-76.5304, -376.6977) (-75.8406, -376.8099) (-74.9891, -376.9957) (-74.1313, -377.1499) (-73.4511, -377.3102) (-72.9654, -377.508) (-72.4977, -377.7435) (-71.915, -378.1285) (-71.4018, -378.6098) (-70.9757, -379.1623) (-70.6032, -379.7528) (-70.2552, -380.5572) (-69.9982, -381.5749) (-69.7828, -383.658) (-69.5247, -386.7848) (-68.9355, -390.9299) (-68.2366, -395.0558) (-67.4057, -399.1577) (-66.4705, -403.237) (-65.7568, -405.9341) (-65.4, -407.2826) knots 0 0 0 0 0.062508 0.125015 0.187523 0.25003 0.312536 0.375043 0.390666 0.406283 0.421892 0.429706 0.437518 0.453124 0.460937 0.468749 0.47656 0.484373 0.5 0.515627 0.52344 0.531251 0.539063 0.546876 0.562482 0.570294 0.578108 0.593717 0.609334 0.624957 0.687464 0.74997 0.812477 0.874985 0.937492 1 1 1 1 projected
  arc A31 (-65.4, -407.2826) -> (-55.644, -408.7297) centre (0, 0) ccw projected
  spline S29 degree 3 poles (-55.644, -408.7297) (-54.9111, -407.5429) (-53.4453, -405.1691) (-51.3661, -401.5369) (-49.3803, -397.8529) (-47.5138, -394.1076) (-45.7467, -390.312) (-44.5921, -387.3947) (-43.7813, -385.4638) (-43.2399, -384.5646) (-42.6733, -383.8958) (-42.1455, -383.4388) (-41.5773, -383.0338) (-40.9465, -382.7222) (-40.2772, -382.5229) (-39.7613, -382.4333) (-39.239, -382.3851) (-38.5416, -382.4291) (-37.676, -382.5305) (-36.8072, -382.5999) (-36.1146, -382.6928) (-35.6118, -382.842) (-35.1232, -383.0305) (-34.5057, -383.3566) (-33.9478, -383.7853) (-33.4695, -384.2933) (-33.041, -384.8445) (-32.6158, -385.611) (-32.2602, -386.5985) (-31.8417, -388.6505) (-31.2784, -391.7369) (-30.2857, -395.8044) (-29.1858, -399.8419) (-27.9568, -403.8425) (-26.6262, -407.8106) (-25.6517, -410.4247) (-25.1644, -411.7317) knots 0 0 0 0 0.062508 0.125015 0.187523 0.25003 0.312536 0.375043 0.390666 0.406283 0.421892 0.429706 0.437518 0.453124 0.460937 0.468749 0.47656 0.484373 0.5 0.515627 0.52344 0.531251 0.539063 0.546876 0.562482 0.570294 0.578108 0.593717 0.609334 0.624957 0.687464 0.74997 0.812477 0.874985 0.937492 1 1 1 1 projected
  arc A32 (-25.1644, -411.7317) -> (-15.3136, -412.2157) centre (0, 0) ccw projected
  spline S30 degree 3 poles (-15.3136, -412.2157) (-14.7005, -410.9627) (-13.4744, -408.4567) (-11.7613, -404.6382) (-10.1461, -400.7772) (-8.6557, -396.867) (-7.2691, -392.9165) (-6.406, -389.9001) (-5.7884, -387.899) (-5.3377, -386.951) (-4.8395, -386.2299) (-4.359, -385.7235) (-3.8332, -385.2647) (-3.236, -384.8928) (-2.5894, -384.6288) (-2.0848, -384.4891) (-1.5698, -384.3899) (-0.8714, -384.3654) (0, -384.3814) (0.8714, -384.3654) (1.5698, -384.3899) (2.0848, -384.4891) (2.5894, -384.6288) (3.236, -384.8928) (3.8332, -385.2647) (4.359, -385.7235) (4.8395, -386.2299) (5.3377, -386.951) (5.7884, -387.899) (6.406, -389.9001) (7.2691, -392.9165) (8.6557, -396.867) (10.1461, -400.7772) (11.7613, -404.6382) (13.4744, -408.4567) (14.7005, -410.9627) (15.3136, -412.2157) knots 0 0 0 0 0.062508 0.125015 0.187523 0.25003 0.312536 0.375043 0.390666 0.406283 0.421892 0.429706 0.437518 0.453124 0.460937 0.468749 0.47656 0.484373 0.5 0.515627 0.52344 0.531251 0.539063 0.546876 0.562482 0.570294 0.578108 0.593717 0.609334 0.624957 0.687464 0.74997 0.812477 0.874985 0.937492 1 1 1 1 projected
  arc A33 (15.3136, -412.2157) -> (25.1644, -411.7317) centre (0, 0) ccw projected
  spline S31 degree 3 poles (25.1644, -411.7317) (25.6517, -410.4247) (26.6262, -407.8106) (27.9568, -403.8425) (29.1858, -399.8419) (30.2857, -395.8044) (31.2784, -391.7369) (31.8417, -388.6505) (32.2602, -386.5985) (32.6158, -385.611) (33.041, -384.8445) (33.4695, -384.2933) (33.9478, -383.7853) (34.5057, -383.3566) (35.1232, -383.0305) (35.6118, -382.842) (36.1146, -382.6928) (36.8072, -382.5999) (37.676, -382.5305) (38.5416, -382.4291) (39.239, -382.3851) (39.7613, -382.4333) (40.2772, -382.5229) (40.9465, -382.7222) (41.5773, -383.0338) (42.1455, -383.4388) (42.6733, -383.8958) (43.2399, -384.5646) (43.7813, -385.4638) (44.5921, -387.3947) (45.7467, -390.312) (47.5138, -394.1076) (49.3803, -397.8529) (51.3661, -401.5369) (53.4453, -405.1691) (54.9111, -407.5429) (55.644, -408.7297) knots 0 0 0 0 0.062508 0.125015 0.187523 0.25003 0.312536 0.375043 0.390666 0.406283 0.421892 0.429706 0.437518 0.453124 0.460937 0.468749 0.47656 0.484373 0.5 0.515627 0.52344 0.531251 0.539063 0.546876 0.562482 0.570294 0.578108 0.593717 0.609334 0.624957 0.687464 0.74997 0.812477 0.874985 0.937492 1 1 1 1 projected
  arc A34 (55.644, -408.7297) -> (65.4, -407.2826) centre (0, 0) ccw projected
  spline S32 degree 3 poles (65.4, -407.2826) (65.7568, -405.9341) (66.4705, -403.237) (67.4057, -399.1577) (68.2366, -395.0558) (68.9355, -390.9299) (69.5247, -386.7848) (69.7828, -383.658) (69.9982, -381.5749) (70.2552, -380.5572) (70.6032, -379.7528) (70.9757, -379.1623) (71.4018, -378.6098) (71.915, -378.1285) (72.4977, -377.7435) (72.9654, -377.508) (73.4511, -377.3102) (74.1313, -377.1499) (74.9891, -376.9957) (75.8406, -376.8099) (76.5304, -376.6977) (77.0548, -376.6945) (77.5771, -376.7331) (78.2627, -376.8658) (78.921, -377.1141) (79.5261, -377.4615) (80.0962, -377.8645) (80.7256, -378.4745) (81.3525, -379.3164) (82.3487, -381.1585) (83.7837, -383.9485) (85.9143, -387.5526) (88.1389, -391.097) (90.4763, -394.5686) (92.9014, -397.9796) (94.5929, -400.1982) (95.4386, -401.3075) knots 0 0 0 0 0.062508 0.125015 0.187523 0.25003 0.312536 0.375043 0.390666 0.406283 0.421892 0.429706 0.437518 0.453124 0.460937 0.468749 0.47656 0.484373 0.5 0.515627 0.52344 0.531251 0.539063 0.546876 0.562482 0.570294 0.578108 0.593717 0.609334 0.624957 0.687464 0.74997 0.812477 0.874985 0.937492 1 1 1 1 projected
  arc A35 (95.4386, -401.3075) -> (105.0057, -398.9111) centre (0, 0) ccw projected
  spline S33 degree 3 poles (105.0057, -398.9111) (105.2286, -397.5341) (105.6745, -394.7801) (106.2054, -390.6287) (106.6303, -386.4651) (106.9214, -382.2906) (107.1015, -378.1077) (107.0519, -374.9707) (107.062, -372.8765) (107.2181, -371.8385) (107.4855, -371.0038) (107.7983, -370.3797) (108.1683, -369.7881) (108.6318, -369.2588) (109.1739, -368.8185) (109.6163, -368.5383) (110.0803, -368.2939) (110.7415, -368.0677) (111.58, -367.8301) (112.4092, -367.5618) (113.0847, -367.3825) (113.6063, -367.3279) (114.1298, -367.3152) (114.8251, -367.38) (115.5046, -367.5626) (116.1409, -367.849) (116.7477, -368.1942) (117.4338, -368.7396) (118.1403, -369.5159) (119.3122, -371.2516) (121.0137, -373.8875) (123.4874, -377.2654) (126.0487, -380.5746) (128.7151, -383.8005) (131.4629, -386.9573) (133.3637, -388.9994) (134.3141, -390.0205) knots 0 0 0 0 0.062508 0.125015 0.187523 0.25003 0.312536 0.375043 0.390666 0.406283 0.421892 0.429706 0.437518 0.453124 0.460937 0.468749 0.47656 0.484373 0.5 0.515627 0.52344 0.531251 0.539063 0.546876 0.562482 0.570294 0.578108 0.593717 0.609334 0.624957 0.687464 0.74997 0.812477 0.874985 0.937492 1 1 1 1 projected
  arc A36 (134.3141, -390.0205) -> (143.6002, -386.6979) centre (0, 0) ccw projected
  spline S34 degree 3 poles (143.6002, -386.6979) (143.6871, -385.3056) (143.8609, -382.5212) (143.9823, -378.3378) (143.9971, -374.1526) (143.8776, -369.9697) (143.6468, -365.7892) (143.2899, -362.6722) (143.0948, -360.5871) (143.1483, -359.5388) (143.3327, -358.6819) (143.5828, -358.0301) (143.893, -357.4051) (144.3024, -356.8329) (144.7987, -356.3416) (145.2115, -356.0194) (145.6494, -355.7307) (146.2852, -355.4408) (147.0964, -355.1221) (147.8953, -354.7738) (148.55, -354.5292) (149.0637, -354.4238) (149.5834, -354.3598) (150.2818, -354.3562) (150.9759, -354.4713) (151.6371, -354.6939) (152.2749, -354.9779) (153.0112, -355.4535) (153.7903, -356.1568) (155.1267, -357.7693) (157.0784, -360.2257) (159.8713, -363.3449) (162.7446, -366.3871) (165.7143, -369.3361) (168.7583, -372.2083) (170.8501, -374.0544) (171.896, -374.9774) knots 0 0 0 0 0.062508 0.125015 0.187523 0.25003 0.312536 0.375043 0.390666 0.406283 0.421892 0.429706 0.437518 0.453124 0.460937 0.468749 0.47656 0.484373 0.5 0.515627 0.52344 0.531251 0.539063 0.546876 0.562482 0.570294 0.578108 0.593717 0.609334 0.624957 0.687464 0.74997 0.812477 0.874985 0.937492 1 1 1 1 projected
  arc A37 (171.896, -374.9774) -> (180.8117, -370.7605) centre (0, 0) ccw projected
  spline S35 degree 3 poles (180.8117, -370.7605) (180.7618, -369.3665) (180.6618, -366.5784) (180.3726, -362.4032) (179.977, -358.2368) (179.4481, -354.0857) (178.8087, -349.948) (178.1481, -346.881) (177.7494, -344.825) (177.7, -343.7765) (177.7995, -342.9057) (177.9845, -342.2325) (178.2319, -341.5801) (178.5833, -340.9705) (179.0291, -340.433) (179.4083, -340.0719) (179.8157, -339.7416) (180.4201, -339.3908) (181.1962, -338.9942) (181.9571, -338.5692) (182.5846, -338.2616) (183.0855, -338.1063) (183.5965, -337.9917) (184.2911, -337.9197) (184.9931, -337.9662) (185.673, -338.1229) (186.3356, -338.3431) (187.1149, -338.7442) (187.9592, -339.3678) (189.4472, -340.8414) (191.6303, -343.0947) (194.7155, -345.9252) (197.8731, -348.6711) (201.1176, -351.3148) (204.4285, -353.8749) (206.6912, -355.5069) (207.8225, -356.323) knots 0 0 0 0 0.062508 0.125015 0.187523 0.25003 0.312536 0.375043 0.390666 0.406283 0.421892 0.429706 0.437518 0.453124 0.460937 0.468749 0.47656 0.484373 0.5 0.515627 0.52344 0.531251 0.539063 0.546876 0.562482 0.570294 0.578108 0.593717 0.609334 0.624957 0.687464 0.74997 0.812477 0.874985 0.937492 1 1 1 1 projected
  arc A38 (207.8225, -356.323) -> (216.282, -351.2526) centre (0, 0) ccw projected
  spline S36 degree 3 poles (216.282, -351.2526) (216.0956, -349.8701) (215.7228, -347.1053) (215.0258, -342.9785) (214.2237, -338.8709) (213.2905, -334.7917) (212.2486, -330.7366) (211.2905, -327.7491) (210.6923, -325.7421) (210.5403, -324.7035) (210.554, -323.8271) (210.6721, -323.139) (210.8544, -322.4655) (211.1443, -321.8245) (211.5353, -321.2458) (211.8773, -320.8492) (212.2504, -320.4807) (212.8174, -320.0722) (213.5509, -319.6015) (214.2665, -319.104) (214.8608, -318.7364) (215.3441, -318.5327) (215.8414, -318.3686) (216.5256, -318.2288) (217.2288, -318.2063) (217.9208, -318.2956) (218.6017, -318.4498) (219.4166, -318.7725) (220.318, -319.3104) (221.9433, -320.6311) (224.3367, -322.6596) (227.6844, -325.174) (231.096, -327.5972) (234.5841, -329.9101) (238.1299, -332.1334) (240.5417, -333.5358) (241.7475, -334.237) knots 0 0 0 0 0.062508 0.125015 0.187523 0.25003 0.312536 0.375043 0.390666 0.406283 0.421892 0.429706 0.437518 0.453124 0.460937 0.468749 0.47656 0.484373 0.5 0.515627 0.52344 0.531251 0.539063 0.546876 0.562482 0.570294 0.578108 0.593717 0.609334 0.624957 0.687464 0.74997 0.812477 0.874985 0.937492 1 1 1 1 projected
  arc A39 (241.7475, -334.237) -> (249.6693, -328.3618) centre (0, 0) ccw projected
  spline S37 degree 3 poles (249.6693, -328.3618) (249.3483, -327.0043) (248.7063, -324.2894) (247.6081, -320.2508) (246.4074, -316.2416) (245.0788, -312.2735) (243.6444, -308.34) (242.3981, -305.4608) (241.6061, -303.5221) (241.353, -302.5034) (241.2807, -301.6299) (241.3308, -300.9336) (241.4462, -300.2454) (241.6719, -299.579) (242.0043, -298.9648) (242.3057, -298.5367) (242.6409, -298.1333) (243.1652, -297.6712) (243.849, -297.1309) (244.5124, -296.5656) (245.0678, -296.1416) (245.5289, -295.8915) (246.0076, -295.6794) (246.6748, -295.4732) (247.3725, -295.3819) (248.0699, -295.403) (248.7627, -295.4896) (249.6053, -295.731) (250.555, -296.1779) (252.3019, -297.3329) (254.8827, -299.117) (258.4607, -301.2912) (262.0934, -303.3684) (265.7913, -305.3283) (269.538, -307.1932) (272.0756, -308.3525) (273.3444, -308.9322) knots 0 0 0 0 0.062508 0.125015 0.187523 0.25003 0.312536 0.375043 0.390666 0.406283 0.421892 0.429706 0.437518 0.453124 0.460937 0.468749 0.47656 0.484373 0.5 0.515627 0.52344 0.531251 0.539063 0.546876 0.562482 0.570294 0.578108 0.593717 0.609334 0.624957 0.687464 0.74997 0.812477 0.874985 0.937492 1 1 1 1 projected
  arc A40 (273.3444, -308.9322) -> (280.6521, -302.3088) centre (0, 0) ccw projected